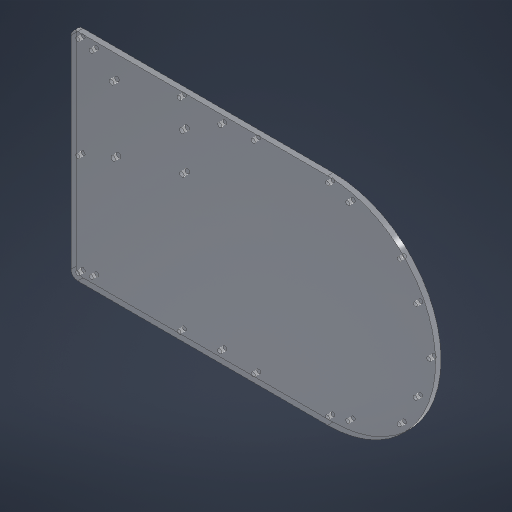
# Autodesk Inventor part: Base_solida_Down
Saved by Autodesk Inventor 2025.2 (Build 292293000, 293)
## iProperties
Created: 2025-04-27
Part Number: Base_solida_Down
Material: Acrilico
Document SubType Name: Modeling
Designer: Tiago
Density: 1.18 g/cm^3
Appearance: Polycarbonate - Clear
Mass: 159.889 g
Surface Area: 836.081 cm^2
Volume: 159.889 cm^3
Author: Tiago
Autodesk Inventor part; units mm, degrees
ref_plane "YZ Plane" through (0, 0, 0) normal (1, 0, 0) x (0, 1, 0)
ref_plane "XZ Plane" through (0, 0, 0) normal (0, 1, 0) x (-1, 0, 0)
ref_plane "XY Plane" through (0, 0, 0) normal (0, 0, 1) x (1, 0, 0)
sketch "Sketch1" plane through (0, 0, 0) normal (0, 0, 1) x (1, 0, 0)
  line L0 (-150, -80) -> (40, -80)
  line L1 (150, -80) -> (150, 80) construction
  line L2 (40, 80) -> (-150, 80)
  line L3 (-150, 80) -> (-150, -80)
  line L4 (-150, -80) -> (150, 80) construction
  line L5 (150, -80) -> (-150, 80) construction
  line L6 (-150, 0) -> (-107, 0) construction
  line L7 (-107, 0) -> (33.79, 0) construction
  line L8 (-7.3128, 0) -> (74.6872, 0) construction
  line L9 (33.6872, 41) -> (74.6872, 41) construction
  line L10 (74.6872, 41) -> (74.6872, 0) construction
  circle A0 centre (74.6872, 41) radius 2 construction
  circle A1 centre (74.6872, -41) radius 2 construction
  circle A2 centre (-7.3128, 41) radius 2 construction
  circle A3 centre (-7.3128, -41) radius 2 construction
  line L11 (150, 0) -> (120, 0) construction
  line L12 (120, 0) -> (120, 0)
  arc A4 (40, -80) -> (120, 0) centre (40, 0) ccw
  arc A5 (120, 0) -> (40, 80) centre (40, 0) ccw
  line L13 (120, 0) -> (115, 0) construction
  circle A6 centre (115, 0) radius 1.5
  line L14 (40, 0) -> (111.7631, 71.7631) construction
  line L15 (96.5685, -56.5685) -> (93.033, -53.033) construction
  circle A7 centre (93.033, -53.033) radius 1.5
  line L16 (40, -80) -> (40, -75) construction
  circle A8 centre (40, -75) radius 1.5
  line L17 (40, -75) -> (-15, -75) construction
  line L18 (-15, -75) -> (-70, -75) construction
  line L19 (-150, -75) -> (-145, -75) construction
  circle A9 centre (-15, -75) radius 1.5
  circle A10 centre (-70, -75) radius 1.5
  circle A11 centre (-145, -75) radius 1.5
  circle A12 centre (-145, 0) radius 1.5
  circle A13 centre (93.033, 53.033) radius 1.5
  circle A14 centre (40, 75) radius 1.5
  circle A15 centre (-15, 75) radius 1.5
  circle A16 centre (-70, 75) radius 1.5
  circle A17 centre (-145, 75) radius 1.5
  line L20 (-145, -80) -> (-145, -75) construction
  line L21 (-150, 0) -> (-145, 0)
  line L22 (120, 0) -> (105, 0) construction
  line L23 (105, -30) -> (105, 30) construction
  circle A18 centre (105, -30) radius 4 construction
  circle A19 centre (105, 30) radius 4 construction
  circle A20 centre (105, -30) radius 1.5
  circle A21 centre (105, 30) radius 1.5
  line L24 (105, 0) -> (55, 0) construction
  line L25 (55, -70) -> (55, 70) construction
  circle A22 centre (55, -70) radius 1.5
  circle A23 centre (55, -70) radius 4 construction
  line L26 (-150, 0) -> (-135, 0) construction
  line L27 (-135, -72.5) -> (-135, 72.5) construction
  circle A24 centre (-135, -72.5) radius 1.5
  circle A25 centre (-135, -72.5) radius 4 construction
  line L28 (-135, 0) -> (-40, 0) construction
  line L29 (-40, -72.5) -> (-40, 72.5) construction
  circle A26 centre (-40, -72.5) radius 4 construction
  circle A27 centre (-40, -72.5) radius 1.5
  circle A28 centre (55, 70) radius 1.5
  circle A29 centre (55, 70) radius 4 construction
  circle A30 centre (-135, 72.5) radius 1.5
  circle A31 centre (-135, 72.5) radius 4 construction
  circle A32 centre (-40, 72.5) radius 4 construction
  circle A33 centre (-40, 72.5) radius 1.5
  line L30 (-150, 60) -> (-120, 60) construction
  line L31 (-120, 80) -> (-120, 60) construction
  circle A34 centre (-120, 60) radius 1.75
  circle A35 centre (-118.73, 11.74) radius 1.75
  line L32 (-120, 60) -> (-67.93, 60) construction
  line L33 (-150, 11.74) -> (-118.73, 11.74) construction
  line L34 (-118.73, 60) -> (-118.73, 11.74) construction
  line L35 (-67.93, 60) -> (-67.93, 54.92) construction
  circle A36 centre (-67.93, 54.92) radius 1.75
  line L36 (-67.93, 54.92) -> (-67.93, 26.98) construction
  circle A37 centre (-67.93, 26.98) radius 1.75
  point P0 (0, 0)
  point P1 (120, -80)
  point P2 (120, 0)
  dimension "d0" = 300
  dimension "d1" = 160
  dimension "d4" = 43
  dimension "d6" = 140.79
  dimension "d9" = 82
  dimension "d11" = 4
  dimension "d47" = 30
  dimension "d49" = 80
  dimension "LF" = 5
  dimension "Furos" = 3
  dimension "d52" = 45
  dimension "d53" = 5
  dimension "d55" = 3
  dimension "d56" = 5
  dimension "d57" = 3
  dimension "d58" = 55
  dimension "d59" = 55
  dimension "d60" = 5
  dimension "d61" = 3
  dimension "d62" = 3
  dimension "d63" = 3
  dimension "d64" = 3
  dimension "d65" = 5
  dimension "d66" = 5
  dimension "d67" = 15
  dimension "d68" = 60
  dimension "d69" = 8
  dimension "d70" = 8
  dimension "d71" = 3
  dimension "FA" = 3
  dimension "d73" = 50
  dimension "d74" = 140
  dimension "d75" = 3
  dimension "AA" = 8
  dimension "d77" = 15
  dimension "d78" = 145
  dimension "d79" = 3
  dimension "d80" = 8
  dimension "d81" = 95
  dimension "d82" = 145
  dimension "d83" = 8
  dimension "d84" = 3
  dimension "d85" = 30
  dimension "d86" = 20
  dimension "d87" = 3.5
  dimension "d89" = 3.5
  dimension "d90" = 52.07
  dimension "d94" = 31.27
  dimension "d95" = 48.26
  dimension "d96" = 5.08
  dimension "d97" = 3.5
  dimension "d98" = 27.94
  dimension "d99" = 3.5
  dimension "d100" = 41
  dimension "d101" = 41
  dimension "d103" = 74.6872
  dimension "d104" = 82
  dimension "d105" = 41
  constraints: 74 end point, 38 centre point, 29 coincident, 16 symmetric about line, 12 horizontal, 11 perpendicular, 11 point on line, 9 midpoint, 5 point on circle, 5 vertical, 4 tangent, 3 equal radius, 3 vertical alignment, 2 horizontal alignment, 2 parallel, 12 other
  measures "d0" distance of L2.end L1.end
  measures "d1" distance of L1.start L1.end
  measures "d4" distance of L6.start L6.end
  measures "d6" distance of L7.start L7.end
  measures "d9" distance of L8.start L8.end
  measures "d11" diameter of A0
  measures "d47" distance of L11.start L11.end
  measures "d49" radius of A4
  measures "LF" distance of L12.end L13.end
  measures "Furos" diameter of A6
  measures "d52" angle of L8 L14
  measures "d53" distance of L15.start L15.end
  measures "d55" diameter of A7
  measures "d56" distance of L0.end L16.end
  measures "d57" diameter of A8
  measures "d58" distance of L17.start L17.end
  measures "d59" distance of L17.end L18.end
  measures "d60" distance of L19.end L19.start
  measures "d61" diameter of A9
  measures "d62" diameter of A10
  measures "d63" diameter of A11
  measures "d64" diameter of A12
  measures "d65" distance of L20.start L19.end
  measures "d66" distance of L6.start L21.end
  measures "d67" distance of L12.end L22.end
  measures "d68" distance of L23.start L23.end
  measures "d69" diameter of A18
  measures "d70" diameter of A19
  measures "d71" diameter of A20
  measures "FA" diameter of A21
  measures "d73" distance of L22.end L24.end
  measures "d74" distance of L25.start L25.end
  measures "d75" diameter of A22
  measures "AA" diameter of A23
  measures "d77" distance of L6.start L26.end
  measures "d78" distance of L27.start L27.end
  measures "d79" diameter of A24
  measures "d80" diameter of A25
  measures "d81" distance of L26.end L28.end
  measures "d82" distance of L29.start L29.end
  measures "d83" diameter of A26
  measures "d84" diameter of A27
  measures "d85" distance of L30.end L30.start
  measures "d86" distance of L31.start L30.end
  measures "d87" diameter of A34
  measures "d89" diameter of A35
  measures "d90" distance of L32.start L32.end
  measures "d94" distance of L33.end L33.start
  measures "d95" distance of L34.start L33.end
  measures "d96" distance of L32.end L35.end
  measures "d97" diameter of A36
  measures "d98" distance of L36.start L36.end
  measures "d99" diameter of A37
  measures "d100" distance of L9.end L8.end
  measures "d101" distance from line of L9.start L10
  measures "d103" distance from line of point (0, 0) L10
  measures "d104" distance of A1.centre A3.centre
  measures "d105" distance from line of L7 A3.centre
extrude "Extrusion1" add sketch "Sketch1" along normal blind 4
fillet "Fillet1" radius 5 2 edges at (-150, -80, 2) (-150, 80, 2)
equation "\"d9\" = L_furos"
equation "\"d53\" = LF"
equation "\"d55\" = Furos"
equation "\"d56\" = LF"
equation "\"d57\" = Furos"
equation "\"d60\" = LF"
equation "\"d61\" = Furos"
equation "\"d62\" = Furos"
equation "\"d63\" = Furos"
equation "\"d64\" = Furos"
equation "\"d65\" = LF"
equation "\"d66\" = LF"
equation "\"d69\" = AA"
equation "\"d70\" = AA"
equation "\"d71\" = FA"
equation "\"d75\" = FA"
equation "\"d79\" = FA"
equation "\"d80\" = AA"
equation "\"d83\" = AA"
equation "\"d84\" = FA"
equation "\"L_furos\" = 82"
body "Solid1"
